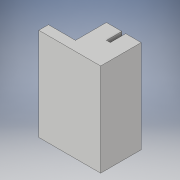
# Autodesk Inventor part: SUspension mounting
Saved by Autodesk Inventor 2018.2 (Build 222227000, 227)
## iProperties
Created: 2018-02-01
Part Number: SUspension mounting
Material: Generic
Document SubType Name: Modeling
Designer: MIABo
Density: 1 g/cm^3
Appearance: Default
Author: MIABo
Autodesk Inventor part; units mm, degrees
ref_plane "YZ Plane" through (0, 0, 0) normal (1, 0, 0) x (0, 1, 0)
ref_plane "XZ Plane" through (0, 0, 0) normal (0, 1, 0) x (-1, 0, 0)
ref_plane "XY Plane" through (0, 0, 0) normal (0, 0, 1) x (1, 0, 0)
sketch "Sketch1" plane through (0, 0, 0) normal (0, 1, 0) x (-1, 0, 0)
  line L0 (-29.8824, 35.8588) -> (-29.8824, 86.6588)
  line L1 (-29.8824, 86.6588) -> (-87.0324, 86.6588)
  line L2 (-87.0324, 86.6588) -> (-87.0324, 35.8588)
  line L3 (-87.0324, 35.8588) -> (-61.6324, 35.8588)
  line L4 (-61.6324, 35.8588) -> (-61.6324, 61.2588)
  line L5 (-61.6324, 61.2588) -> (-55.2824, 61.2588)
  line L6 (-55.2824, 61.2588) -> (-55.2824, 35.8588)
  line L7 (-55.2824, 35.8588) -> (-29.8824, 35.8588)
  line L8 (-29.8824, 86.6588) -> (14.5676, 86.6588)
  line L9 (14.5676, 86.6588) -> (14.5676, 102.4696)
  line L10 (14.5676, 102.4696) -> (-87.0324, 102.4696)
  line L11 (-87.0324, 102.4696) -> (-87.0324, 86.6588)
  point P0 (0, 0)
  dimension "d0" = 25.4
  dimension "d1" = 25.4
  dimension "d2" = 6.35
  dimension "d3" = 50.8
  dimension "d4" = 25.4
  dimension "d5" = 101.6
  constraints: 24 end point, 10 perpendicular, 1 horizontal, 1 point on line, 1 vertical
  measures "d0" distance of L6.end L0.start
  measures "d1" distance of L2.end L3.end
  measures "d2" distance of L4.end L5.end
  measures "d3" distance of L1.end L2.end
  measures "d4" distance of L3.end L4.end
  measures "d5" distance of L9.end L10.end
extrude "Extrusion1" add sketch "Sketch1" along normal blind 152.4
body "Solid1"
